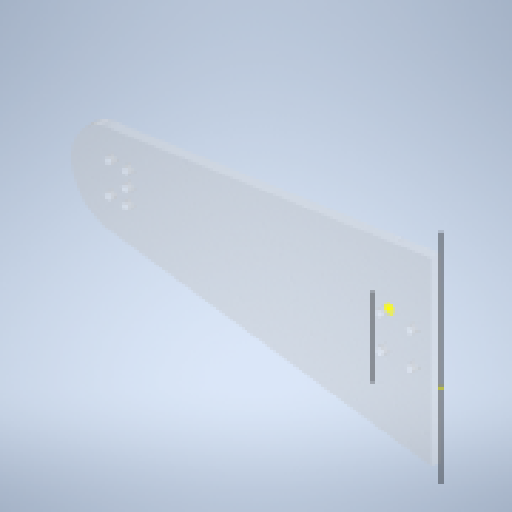
# Autodesk Inventor part: BaseParal
Saved by Autodesk Inventor 2023.1 (Build 271208000, 208)
## iProperties
Created: 2023-05-03
Part Number: BaseParal
Material: Acrylic
Document SubType Name: Modeling
Designer: felip
Density: 1.188 g/cm^3
Appearance: Transparent - Clear
Author: felip
Autodesk Inventor part; units mm, degrees
ref_plane "YZ Plane" through (0, 0, 0) normal (1, 0, 0) x (0, 1, 0)
ref_plane "XZ Plane" through (0, 0, 0) normal (0, 1, 0) x (-1, 0, 0)
ref_plane "XY Plane" through (0, 0, 0) normal (0, 0, 1) x (1, 0, 0)
sketch "Sketch1" plane through (0, 0, 0) normal (0, 0, 1) x (1, 0, 0)
  line L0 (0, -45.5) -> (0, 74.5) projected
  line L1 (0, -35.5) -> (0, 64.5)
  arc A0 (-175, 38.3279) -> (-175, -11.6721) centre (-175, 13.3279) ccw
  line L2 (-175, -11.6721) -> (0, -35.5)
  line L3 (-175, 38.3279) -> (0, 64.5)
  circle A1 centre (-179.5, 4.5) radius 2 projected
  circle A2 centre (-179.5, 21.5) radius 2 projected
  circle A3 centre (-170, 21.5) radius 2 projected
  circle A4 centre (-170, 4.5) radius 2 projected
  circle A5 centre (-170, 13) radius 2 projected
  circle A6 centre (-28.875, 23.65) radius 2 projected
  circle A7 centre (-28.875, 5.35) radius 2 projected
  circle A8 centre (-12.375, 5.35) radius 2 projected
  circle A9 centre (-12.375, 23.65) radius 2 projected
  point P0 (-12.375, 14.5)
  point P1 (0, 29)
  dimension "d0" = 100
  dimension "d1" = 50
  dimension "d2" = 50
  dimension "d3" = 175
  constraints: 6 end point, 2 point on circle, 2 point on line, 1 centre point
  measures "d0" distance of L1.end L1.start
  measures "d1" vertical distance of L1.start point (-12.375, 14.5)
  measures "d2" diameter of A0
  measures "d3" horizontal distance of L1.start A0.centre
extrude "Extrusion1" add sketch "Sketch1" along normal blind 5
sketch "Sketch2" plane through (0, 0, 0) normal (0, 0, -1) x (-1, 0, 0)
  circle A0 centre (28.875, 23.65) radius 2 projected
  line L0 (0, 74.5) -> (0, -45.5)
  line L1 (38, -15.9446) -> (38, 27.4554)
  circle A1 centre (41.4, 23.65) radius 1.5
  circle A2 centre (41.4, -12.95) radius 1.5
  line L2 (59.6, 45.3727) -> (59.6, -35.5339) construction
  circle A3 centre (77.8, 23.65) radius 1.5
  circle A4 centre (77.8, -12.95) radius 1.5
  point P0 (0, 0)
  dimension "d7" = 3.4
  dimension "d8" = 3
  dimension "d9" = 0
  dimension "d10" = 3
  dimension "d11" = 36.6
  dimension "d12" = 21.6
  constraints: 6 end point, 4 centre point, 2 symmetric about line, 2 vertical, 1 parallel, 6 other
  measures "d7" distance from line of L1 A1.centre
  measures "d8" diameter of A1
  measures "d9" vertical distance of A1.centre A0.centre
  measures "d10" diameter of A2
  measures "d11" distance of A1.centre A2.centre
  measures "d12" distance between parallel lines of L1 L2
hole "Hole1" at (-41.4, -12.95, 0) at (-41.4, 23.65, 0) at (-77.8, 23.65, 0) at (-77.8, -12.95, 0) direction (0, 0, 1) diameter 3 end through all
equation "\"d1\" = 0.5 * d0"
body "Solid1"
